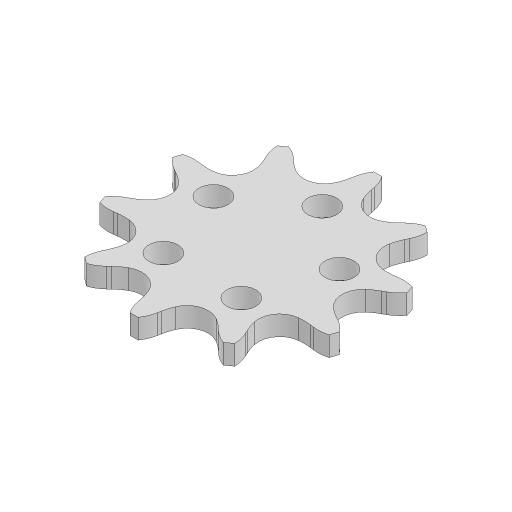
# Autodesk Inventor part: DelrinSprocket
Saved by Autodesk Inventor 2023 (Build 270158000, 158)
## iProperties
Created: 2022-11-17
Part Number: DelrinSprocket
Material: Generic
Document SubType Name: Modeling
Designer: deli
Density: 1 g/cm^3
Appearance: Default
Author: deli
Autodesk Inventor part; units mm, degrees
ref_plane "YZ Plane" through (0, 0, 0) normal (1, 0, 0) x (0, 1, 0)
ref_plane "XZ Plane" through (0, 0, 0) normal (0, 1, 0) x (-1, 0, 0)
ref_plane "XY Plane" through (0, 0, 0) normal (0, 0, 1) x (1, 0, 0)
sketch "Sketch1" plane through (0, 0, 0) normal (0, 1, 0) x (-1, 0, 0)
  spline S0 degree 3 poles (1.65216, 11.314136) (1.711701, 11.173866) (1.783918, 11.038672) (1.931129, 10.814592) (2.000274, 10.72338) (2.075186, 10.63722) knots 0 0 0 0 0.57299817 0.57299817 1 1 1 1
  arc A0 (2.075186, 10.63722) -> (4.573541, 9.825455) centre (4, 12.310734) ccw
  spline S1 degree 3 poles (4.573541, 9.825455) (4.717404, 9.858655) (4.858319, 9.904332) (5.105099, 10.008843) (5.211649, 10.063151) (5.313656, 10.124443) knots 0 0 0 0 0.55246567 0.55246567 1 1 1 1
  spline S2 degree 3 poles (5.313656, 10.124443) (5.51151, 10.243326) (5.703375, 10.372834) (6.083521, 10.660028) (6.267566, 10.816194) (6.440683, 10.979903) knots 0 0 0 0 0.48705824 0.48705824 1 1 1 1
  spline S3 degree 3 poles (6.752179, 11.27447) (6.823505, 11.34192) (6.896966, 11.406693) (7.358577, 11.786242) (7.788733, 12.02573) (8.239696, 12.186595) knots 0 0 0 0 0.16340683 0.16340683 1 1 1 1
  ellipse E0 centre (5.037782, 9.654937) end of major axis (11.199924, 15.481756) minor radius 0.001189 (6.440683, 10.979903) -> (6.752179, 11.27447) ccw
  arc A1 (9.043935, 11.602282) -> (8.239696, 12.186595) centre (0, 0) ccw
  spline S4 degree 3 poles (9.043935, 11.602282) (9.038734, 11.419764) (9.021711, 11.236678) (8.929899, 10.66235) (8.811576, 10.275215) (8.63612, 9.905707) knots 0 0 0 0 0.31776377 0.31776377 1 1 1 1
  ellipse E1 centre (7.62563, 7.774755) end of major axis (3.988202, 0.113624) minor radius 0.001189 (8.63612, 9.905707) -> (8.452228, 9.51843) ccw
  spline S5 degree 3 poles (8.452228, 9.51843) (8.252479, 9.09776) (8.095159, 8.651102) (7.986908, 8.182212) knots 0 0 0 0 1 1 1 1
  spline S6 degree 3 poles (7.986908, 8.182212) (7.952629, 8.033734) (7.931589, 7.881912) (7.918974, 7.614099) (7.921301, 7.499665) (7.931261, 7.385928) knots 0 0 0 0 0.57299817 0.57299817 1 1 1 1
  arc A2 (7.931261, 7.385928) -> (9.47533, 5.260701) centre (10.472136, 7.608452) ccw
  spline S7 degree 3 poles (9.47533, 5.260701) (9.611232, 5.202999) (9.752083, 5.157125) (10.013162, 5.096622) (10.131285, 5.07793) (10.249837, 5.067558) knots 0 0 0 0 0.55246567 0.55246567 1 1 1 1
  spline S8 degree 3 poles (10.249837, 5.067558) (10.479781, 5.04744) (10.711126, 5.039439) (11.187478, 5.04834) (11.428167, 5.066502) (11.664447, 5.09719) knots 0 0 0 0 0.48705824 0.48705824 1 1 1 1
  ellipse E2 centre (9.750681, 4.849874) end of major axis (18.160877, 5.941854) minor radius 0.001189 (11.664447, 5.09719) -> (12.089595, 5.152407) ccw
  spline S9 degree 3 poles (12.089595, 5.152407) (12.186945, 5.16505) (12.284449, 5.174273) (12.880993, 5.210007) (13.369764, 5.150917) (13.829155, 5.015991) knots 0 0 0 0 0.16340683 0.16340683 1 1 1 1
  arc A3 (14.136347, 4.070552) -> (13.829155, 5.015991) centre (0, 0) ccw
  spline S10 degree 3 poles (14.136347, 4.070552) (14.024859, 3.925949) (13.903471, 3.787835) (13.491612, 3.377159) (13.168334, 3.133509) (12.809196, 2.937701) knots 0 0 0 0 0.31776377 0.31776377 1 1 1 1
  ellipse E3 centre (10.739151, 1.807676) end of major axis (3.29331, -2.252282) minor radius 0.001189 (12.809196, 2.937701) -> (12.432789, 2.732477) ccw
  spline S11 degree 3 poles (12.432789, 2.732477) (12.023925, 2.509557) (11.634112, 2.240673) (11.270928, 1.924962) knots 0 0 0 0 1 1 1 1
  spline S12 degree 3 poles (11.270928, 1.924962) (11.155922, 1.82499) (11.049661, 1.71453) (10.88204, 1.50528) (10.81666, 1.411333) (10.757865, 1.313463) knots 0 0 0 0 0.57299817 0.57299817 1 1 1 1
  arc A4 (10.757865, 1.313463) -> (10.757865, -1.313463) centre (12.944272, 0) ccw
  spline S13 degree 3 poles (10.757865, -1.313463) (10.833896, -1.440025) (10.920883, -1.559929) (11.096538, -1.762335) (11.181114, -1.846888) (11.270928, -1.924962) knots 0 0 0 0 0.55246567 0.55246567 1 1 1 1
  spline S14 degree 3 poles (11.270928, -1.924962) (11.445132, -2.076395) (11.627591, -2.21885) (12.0182, -2.491642) (12.223596, -2.618421) (12.432789, -2.732477) knots 0 0 0 0 0.48705824 0.48705824 1 1 1 1
  ellipse E4 centre (10.739151, -1.807676) end of major axis (18.184992, -5.867635) minor radius 0.001189 (12.432789, -2.732477) -> (12.809196, -2.937701) ccw
  spline S15 degree 3 poles (12.809196, -2.937701) (12.895386, -2.984693) (12.979689, -3.034543) (13.483307, -3.356273) (13.844, -3.691371) (14.136347, -4.070552) knots 0 0 0 0 0.16340683 0.16340683 1 1 1 1
  arc A5 (13.829155, -5.015991) -> (14.136347, -4.070552) centre (0, 0) ccw
  spline S16 degree 3 poles (13.829155, -5.015991) (13.653964, -5.067446) (13.474578, -5.107832) (12.899988, -5.197992) (12.495237, -5.20509) (12.089595, -5.152407) knots 0 0 0 0 0.31776377 0.31776377 1 1 1 1
  ellipse E5 centre (9.750681, -4.849874) end of major axis (1.340485, -3.757893) minor radius 0.001189 (12.089595, -5.152407) -> (11.664447, -5.09719) ccw
  spline S17 degree 3 poles (11.664447, -5.09719) (11.202641, -5.037212) (10.729229, -5.025617) (10.249837, -5.067558) knots 0 0 0 0 1 1 1 1
  spline S18 degree 3 poles (10.249837, -5.067558) (10.098033, -5.080839) (9.947139, -5.107744) (9.688536, -5.178506) (9.580422, -5.21608) (9.47533, -5.260701) knots 0 0 0 0 0.57299817 0.57299817 1 1 1 1
  arc A6 (9.47533, -5.260701) -> (7.931261, -7.385928) centre (10.472136, -7.608452) ccw
  spline S19 degree 3 poles (7.931261, -7.385928) (7.91838, -7.533009) (7.918277, -7.681143) (7.941413, -7.94814) (7.960137, -8.066258) (7.986908, -8.182212) knots 0 0 0 0 0.55246567 0.55246567 1 1 1 1
  spline S20 degree 3 poles (7.986908, -8.182212) (8.038831, -8.407119) (8.102711, -8.629614) (8.258377, -9.079902) (8.350028, -9.303197) (8.452228, -9.51843) knots 0 0 0 0 0.48705824 0.48705824 1 1 1 1
  ellipse E6 centre (7.62563, -7.774755) end of major axis (11.263058, -15.435886) minor radius 0.001189 (8.452228, -9.51843) -> (8.63612, -9.905707) ccw
  spline S21 degree 3 poles (8.63612, -9.905707) (8.678228, -9.994385) (8.71713, -10.084266) (8.935457, -10.640571) (9.030298, -11.123681) (9.043935, -11.602282) knots 0 0 0 0 0.16340683 0.16340683 1 1 1 1
  arc A7 (8.239696, -12.186595) -> (9.043935, -11.602282) centre (0, 0) ccw
  spline S22 degree 3 poles (8.239696, -12.186595) (8.067719, -12.125248) (7.898854, -12.052481) (7.381007, -11.787686) (7.049383, -11.555522) (6.752179, -11.27447) knots 0 0 0 0 0.31776377 0.31776377 1 1 1 1
  spline S23 degree 3 poles (6.440683, -10.979903) (6.320723, -10.866463) (6.195025, -10.756181) (5.826711, -10.457786) (5.576398, -10.282314) (5.313656, -10.124443) knots 0 0 0 0 0.35725077 0.35725077 1 1 1 1
  spline S24 degree 3 poles (5.313656, -10.124443) (5.183038, -10.04596) (5.045148, -9.979034) (4.794341, -9.884278) (4.684789, -9.851129) (4.573541, -9.825455) knots 0 0 0 0 0.57299817 0.57299817 1 1 1 1
  arc A8 (4.573541, -9.825455) -> (2.075186, -10.63722) centre (4, -12.310734) ccw
  ellipse E7 centre (5.037782, -9.654937) end of major axis (-1.124359, -3.828117) minor radius 0.001189 (6.752179, -11.27447) -> (6.440683, -10.979903) ccw
  spline S25 degree 3 poles (2.075186, -10.63722) (1.978312, -10.74864) (1.891158, -10.868421) (1.752939, -11.098026) (1.698659, -11.204591) (1.65216, -11.314135) knots 0 0 0 0 0.55246567 0.55246567 1 1 1 1
  spline S26 degree 3 poles (1.65216, -11.314135) (1.561971, -11.526609) (1.482871, -11.744158) (1.344135, -12.199947) (1.287032, -12.434468) (1.243203, -12.668667) knots 0 0 0 0 0.48705824 0.48705824 1 1 1 1
  ellipse E8 centre (1.599378, -10.772142) end of major axis (0.039019, -19.108154) minor radius 0.001189 (1.243203, -12.668667) -> (1.16434, -13.090069) ccw
  spline S27 degree 3 poles (1.16434, -13.090069) (1.146282, -13.186562) (1.124923, -13.282143) (0.974566, -13.860533) (0.767329, -14.307123) (0.497047, -14.702335) knots 0 0 0 0 0.16340683 0.16340683 1 1 1 1
  arc A9 (-0.497047, -14.702335) -> (0.497047, -14.702335) centre (0, 0) ccw
  spline S28 degree 3 poles (-0.497047, -14.702335) (-0.600121, -14.551618) (-0.693964, -14.393492) (-0.957268, -13.874885) (-1.089095, -13.492138) (-1.16434, -13.090069) knots 0 0 0 0 0.31776377 0.31776377 1 1 1 1
  ellipse E9 centre (-1.599378, -10.772142) end of major axis (-3.159736, -2.43613) minor radius 0.001189 (-1.16434, -13.090069) -> (-1.243203, -12.668667) ccw
  spline S29 degree 3 poles (-1.243203, -12.668667) (-1.328867, -12.210928) (-1.464131, -11.757104) (-1.65216, -11.314135) knots 0 0 0 0 1 1 1 1
  spline S30 degree 3 poles (-1.65216, -11.314135) (-1.711701, -11.173866) (-1.783918, -11.038671) (-1.931129, -10.814592) (-2.000274, -10.72338) (-2.075186, -10.63722) knots 0 0 0 0 0.57299817 0.57299817 1 1 1 1
  arc A10 (-2.075186, -10.63722) -> (-4.573541, -9.825455) centre (-4, -12.310734) ccw
  spline S31 degree 3 poles (-4.573541, -9.825455) (-4.717404, -9.858655) (-4.858319, -9.904332) (-5.105099, -10.008843) (-5.211649, -10.063151) (-5.313656, -10.124443) knots 0 0 0 0 0.55246567 0.55246567 1 1 1 1
  spline S32 degree 3 poles (-5.313656, -10.124443) (-5.72113, -10.369278) (-6.098145, -10.655981) (-6.440683, -10.979903) knots 0 0 0 0 1 1 1 1
  ellipse E10 centre (-5.037782, -9.654937) end of major axis (-11.199924, -15.481756) minor radius 0.001189 (-6.440683, -10.979903) -> (-6.752179, -11.27447) ccw
  spline S33 degree 3 poles (-6.752179, -11.27447) (-6.823505, -11.34192) (-6.896966, -11.406693) (-7.358577, -11.786242) (-7.788733, -12.02573) (-8.239696, -12.186595) knots 0 0 0 0 0.16340683 0.16340683 1 1 1 1
  arc A11 (-9.043935, -11.602282) -> (-8.239696, -12.186595) centre (0, 0) ccw
  spline S34 degree 3 poles (-9.043935, -11.602282) (-9.038734, -11.419764) (-9.021711, -11.236678) (-8.929899, -10.66235) (-8.811576, -10.275215) (-8.63612, -9.905707) knots 0 0 0 0 0.31776377 0.31776377 1 1 1 1
  ellipse E11 centre (-7.62563, -7.774755) end of major axis (-3.988202, -0.113624) minor radius 0.001189 (-8.63612, -9.905707) -> (-8.452228, -9.51843) ccw
  spline S35 degree 3 poles (-8.452228, -9.51843) (-8.252479, -9.09776) (-8.095159, -8.651102) (-7.986908, -8.182212) knots 0 0 0 0 1 1 1 1
  spline S36 degree 3 poles (-7.986908, -8.182212) (-7.952629, -8.033734) (-7.931589, -7.881912) (-7.918974, -7.614099) (-7.921301, -7.499665) (-7.931261, -7.385928) knots 0 0 0 0 0.57299817 0.57299817 1 1 1 1
  arc A12 (-7.931261, -7.385928) -> (-9.47533, -5.260701) centre (-10.472136, -7.608452) ccw
  spline S37 degree 3 poles (-9.47533, -5.260701) (-9.611232, -5.202999) (-9.752083, -5.157125) (-10.013162, -5.096622) (-10.131285, -5.07793) (-10.249837, -5.067558) knots 0 0 0 0 0.55246567 0.55246567 1 1 1 1
  spline S38 degree 3 poles (-10.249837, -5.067558) (-10.479781, -5.04744) (-10.711126, -5.039439) (-11.187478, -5.04834) (-11.428167, -5.066502) (-11.664447, -5.09719) knots 0 0 0 0 0.48705824 0.48705824 1 1 1 1
  ellipse E12 centre (-9.750681, -4.849874) end of major axis (-18.160877, -5.941854) minor radius 0.001189 (-11.664447, -5.09719) -> (-12.089595, -5.152407) ccw
  spline S39 degree 3 poles (-12.089595, -5.152407) (-12.186945, -5.16505) (-12.284449, -5.174273) (-12.880993, -5.210007) (-13.369764, -5.150917) (-13.829155, -5.015991) knots 0 0 0 0 0.16340683 0.16340683 1 1 1 1
  arc A13 (-14.136347, -4.070552) -> (-13.829155, -5.015991) centre (0, 0) ccw
  spline S40 degree 3 poles (-14.136347, -4.070552) (-14.024859, -3.925949) (-13.903471, -3.787835) (-13.491612, -3.377159) (-13.168334, -3.133509) (-12.809196, -2.937701) knots 0 0 0 0 0.31776377 0.31776377 1 1 1 1
  ellipse E13 centre (-10.739151, -1.807676) end of major axis (-3.29331, 2.252282) minor radius 0.001189 (-12.809196, -2.937701) -> (-12.432789, -2.732477) ccw
  spline S41 degree 3 poles (-12.432789, -2.732477) (-12.023925, -2.509557) (-11.634112, -2.240673) (-11.270928, -1.924962) knots 0 0 0 0 1 1 1 1
  spline S42 degree 3 poles (-11.270928, -1.924962) (-11.155922, -1.82499) (-11.049661, -1.71453) (-10.88204, -1.50528) (-10.81666, -1.411333) (-10.757865, -1.313463) knots 0 0 0 0 0.57299817 0.57299817 1 1 1 1
  arc A14 (-10.757865, -1.313463) -> (-10.757865, 1.313463) centre (-12.944272, 0) ccw
  spline S43 degree 3 poles (-11.270928, 1.924962) (-11.445132, 2.076395) (-11.627591, 2.21885) (-12.0182, 2.491642) (-12.223596, 2.618421) (-12.432789, 2.732477) knots 0 0 0 0 0.48705824 0.48705824 1 1 1 1
  spline S44 degree 3 poles (-10.757865, 1.313463) (-10.833896, 1.440025) (-10.920883, 1.559929) (-11.096538, 1.762335) (-11.181114, 1.846888) (-11.270928, 1.924962) knots 0 0 0 0 0.55246567 0.55246567 1 1 1 1
  spline S45 degree 3 poles (-12.809196, 2.937701) (-12.895386, 2.984693) (-12.979689, 3.034543) (-13.483307, 3.356273) (-13.844, 3.691371) (-14.136347, 4.070552) knots 0 0 0 0 0.16340683 0.16340683 1 1 1 1
  ellipse E14 centre (-10.739151, 1.807676) end of major axis (-18.184992, 5.867635) minor radius 0.001189 (-12.432789, 2.732477) -> (-12.809196, 2.937701) ccw
  arc A15 (-13.829155, 5.015991) -> (-14.136347, 4.070552) centre (0, 0) ccw
  spline S46 degree 3 poles (-13.829155, 5.015991) (-13.653964, 5.067446) (-13.474578, 5.107832) (-12.899988, 5.197992) (-12.495237, 5.20509) (-12.089595, 5.152407) knots 0 0 0 0 0.31776377 0.31776377 1 1 1 1
  ellipse E15 centre (-9.750681, 4.849874) end of major axis (-1.340485, 3.757893) minor radius 0.001189 (-12.089595, 5.152407) -> (-11.664446, 5.09719) ccw
  spline S47 degree 3 poles (-11.664446, 5.09719) (-11.202637, 5.037211) (-10.729229, 5.025617) (-10.249837, 5.067558) knots 0 0 0 0 1 1 1 1
  spline S48 degree 3 poles (-10.249837, 5.067558) (-10.098033, 5.080839) (-9.947139, 5.107744) (-9.688536, 5.178506) (-9.580422, 5.21608) (-9.47533, 5.260701) knots 0 0 0 0 0.57299817 0.57299817 1 1 1 1
  arc A16 (-9.47533, 5.260701) -> (-7.931261, 7.385928) centre (-10.472136, 7.608452) ccw
  spline S49 degree 3 poles (-7.931261, 7.385928) (-7.91838, 7.533009) (-7.918277, 7.681143) (-7.941413, 7.94814) (-7.960137, 8.066258) (-7.986908, 8.182212) knots 0 0 0 0 0.55246567 0.55246567 1 1 1 1
  spline S50 degree 3 poles (-7.986908, 8.182212) (-8.038831, 8.407119) (-8.102711, 8.629614) (-8.258377, 9.079902) (-8.350028, 9.303197) (-8.452228, 9.51843) knots 0 0 0 0 0.48705824 0.48705824 1 1 1 1
  ellipse E16 centre (-7.62563, 7.774755) end of major axis (-11.263058, 15.435886) minor radius 0.001189 (-8.452228, 9.51843) -> (-8.63612, 9.905707) ccw
  spline S51 degree 3 poles (-8.63612, 9.905707) (-8.678228, 9.994385) (-8.71713, 10.084266) (-8.935457, 10.640571) (-9.030298, 11.123681) (-9.043935, 11.602282) knots 0 0 0 0 0.16340683 0.16340683 1 1 1 1
  arc A17 (-8.239696, 12.186595) -> (-9.043935, 11.602282) centre (0, 0) ccw
  spline S52 degree 3 poles (-8.239696, 12.186595) (-8.067719, 12.125248) (-7.898854, 12.052481) (-7.381007, 11.787686) (-7.049383, 11.555522) (-6.752179, 11.27447) knots 0 0 0 0 0.31776377 0.31776377 1 1 1 1
  ellipse E17 centre (-5.037782, 9.654937) end of major axis (1.124359, 3.828117) minor radius 0.001189 (-6.752179, 11.27447) -> (-6.440683, 10.979903) ccw
  spline S53 degree 3 poles (-6.440683, 10.979903) (-6.102328, 10.659937) (-5.726145, 10.372292) (-5.313656, 10.124443) knots 0 0 0 0 1 1 1 1
  spline S54 degree 3 poles (-5.313656, 10.124443) (-5.183038, 10.04596) (-5.045148, 9.979034) (-4.794341, 9.884278) (-4.684789, 9.851129) (-4.573541, 9.825455) knots 0 0 0 0 0.57299817 0.57299817 1 1 1 1
  arc A18 (-4.573541, 9.825455) -> (-2.075186, 10.63722) centre (-4, 12.310734) ccw
  spline S55 degree 3 poles (-2.075186, 10.63722) (-1.978312, 10.74864) (-1.891158, 10.868421) (-1.752939, 11.098026) (-1.698659, 11.204591) (-1.65216, 11.314135) knots 0 0 0 0 0.55246567 0.55246567 1 1 1 1
  spline S56 degree 3 poles (-1.65216, 11.314135) (-1.561971, 11.526609) (-1.482871, 11.744158) (-1.344135, 12.199947) (-1.287032, 12.434468) (-1.243203, 12.668667) knots 0 0 0 0 0.48705824 0.48705824 1 1 1 1
  ellipse E18 centre (-1.599378, 10.772142) end of major axis (-0.039019, 19.108154) minor radius 0.001189 (-1.243203, 12.668667) -> (-1.16434, 13.090069) ccw
  spline S57 degree 3 poles (-1.16434, 13.090069) (-1.146282, 13.186562) (-1.124923, 13.282143) (-0.974566, 13.860533) (-0.767329, 14.307123) (-0.497047, 14.702335) knots 0 0 0 0 0.16340683 0.16340683 1 1 1 1
  arc A19 (0.497047, 14.702335) -> (-0.497047, 14.702335) centre (0, 0) ccw
  spline S58 degree 3 poles (0.497047, 14.702335) (0.600121, 14.551618) (0.693964, 14.393492) (0.957268, 13.874885) (1.089095, 13.492138) (1.16434, 13.090069) knots 0 0 0 0 0.31776377 0.31776377 1 1 1 1
  ellipse E19 centre (1.599378, 10.772142) end of major axis (3.159736, 2.43613) minor radius 0.001189 (1.16434, 13.090069) -> (1.243203, 12.668667) ccw
  spline S59 degree 3 poles (1.243203, 12.668667) (1.328867, 12.210928) (1.464131, 11.757104) (1.65216, 11.314136) knots 0 0 0 0 1 1 1 1
  point P0 (-50.988834, -24.630484)
  constraints: 40 point on circle, 20 centre point, 260 other
extrude "Extrusion1" add sketch "Sketch1" along normal blind 2.38125
sketch "Sketch2" plane through (0, 2.38125, 0) normal (0, 1, 0) x (1, 0, 0)
  circle A0 centre (0, 0) radius 8 construction
  circle A1 centre (0, 8) radius 1.75
  circle A2 centre (7.608452, 2.472136) radius 1.75
  circle A3 centre (4.702282, -6.472136) radius 1.75
  circle A4 centre (-4.702282, -6.472136) radius 1.75
  circle A5 centre (-7.608452, 2.472136) radius 1.75
  line L0 (0, 8) -> (0, 0) construction
  dimension "d2" = 3.5
  dimension "d3" = 16
  dimension "d4" = 72
  dimension "d5" = 72
  dimension "d6" = 72
  dimension "d7" = 72
  constraints: 6 centre point, 5 point on circle, 4 equal radius, 2 end point, 1 coincident, 1 vertical
  measures "d2" diameter of A1
  measures "d3" diameter of A0
extrude "Extrusion2" cut sketch "Sketch2" against normal blind 2.38125
equation "\"d5\" = d4"
equation "\"d6\" = d5"
equation "\"d7\" = d6"
body "Solid1"
